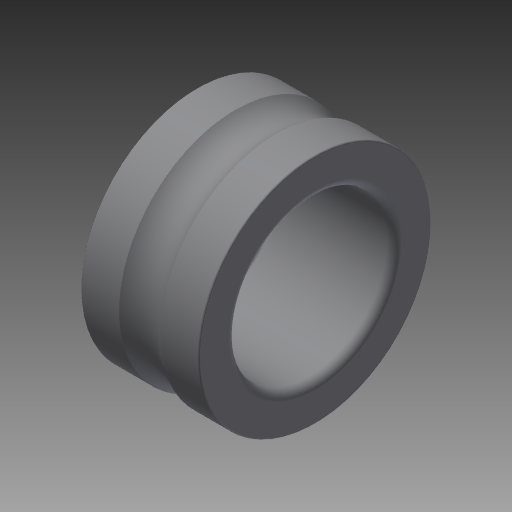
# Autodesk Inventor part: W 637/4 X_PART1
Saved by Autodesk Inventor 2019.1 (Build 231200000, 200)
## iProperties
Category: PARTsolutions
Company: SKF
Created: 2018-08-12
Part Number: W 637/4 X_PART1
Material: Allgemein
Catalog Web Link: www.cadenas.de
Description: -Deep groove ball bearings, stainless steel, single row
Vendor: SKF
Document SubType Name: Modeling
Designer: psadmin
Manufacturer: SKF
Mass: 0.0415935 g
Surface Area: 1.2092 cm^2
Volume: 0.0415935 cm^3
Density: 1 g/cm^3
Appearance: PSOLRGB-175-175-175
PSOL_IDENT_0: {$CADENAS_DATA\23d-libs\skf\bearings_units_and_housings\ball_bearings\deep_groove_ball_bearings\deep
PSOL_IDENT_1: _groove_ball_bearings_stainless_steel\bb1_004_104.prj},197 {VTYP=3D},{NB=W 637/4 X_PART1},{LINA=W 63
PSOL_IDENT_2: 7/4 X_PART1},{NN=BB1_004_104_PART1},{NOPRJ=TRUE},{DATE=13.07.2018 14:28:03},{GEOMDATE=26.07.2017 12:
PSOL_IDENT_3: 34:56},{VERSION=},{LINEID=77360},{WBVAR=},{WBNUMERIC=}  {NB=W 637/4 X_PART1},{LINA=W 637/4 X_PART1},
PSOL_IDENT_4: {KT=DUMMY},{PRODUCTID=},{DESIGNATION=W 637/4 X},{DD=4.000},{D=10.000},{B=3.000},{DD1=5.900},{DD2=MIN
PSOL_IDENT_5: },{D1=8.200},{D2=MIN},{R12A=0.200},{LOAD1=0.553},{LOAD2=0.245},{LOAD3=0.011},{SPEED1=80000},{SPEED2=
PSOL_IDENT_6: },{MASS=0.001},{PITCH=7.100},{DW=1.588},{Z=8.000},{II=1.000},{TYPEID=MIN},{YALG=2.95},{HALG=0.95},{H
PSOL_IDENT_7: ELP=0.9},{HELP2=500000007523733109938344427520},{YALG1=4.1},{HALG1=0.9},{TAXONOMY=2},{DESIGN=dgbbw},
PSOL_IDENT_8: {MAPPING=BCZ50,DESIGNATION|IRD01,DD|ORD10,D|BCW30,B|IRD30,DD1|ORD30,D1|ORD43,D2|IRD43,DD2|ORR20,R12A
PSOL_IDENT_9: |BCC02,LOAD1|BCC16,LOAD2|BCC12,LOAD3|BCC45,SPEED1|BCM01,MASS|BCD50,PITCH|RBD10,DW|BCN81,Z|BCN80,II},
PSOL_IDENT_10: {DESIGNLIST=dgbbw2z,dgbbw,dgbbw2rs},{SH=2.95},{SORT=DD},{RHELP=500000007523733109938344427520},{PIM=
PSOL_IDENT_11: W 637/4 X},{R12=0.2},{HIDE=MIN}
NT: Deep groove ball bearings, stainless steel, single row
NB: W 637/4 X_PART1
NBSYN: $DESIGNATION._PART1
LINA: W 637/4 X_PART1
SUPPLIER: SKF
ARTICLENO: W 637/4 X_PART1
BOMINFO: W 637/4 X_PART1
CREATOR: CADENAS GmbH
Title: W 637/4 X_PART1
Author: Cadenas PARTsolutions
Comments: Deep groove ball bearings, stainless steel, single row
Autodesk Inventor part; units mm, degrees
ref_plane "YZ Plane" through (0, 0, 0) normal (1, 0, 0) x (0, 1, 0)
ref_plane "XZ Plane" through (0, 0, 0) normal (0, 1, 0) x (-1, 0, 0)
ref_plane "XY Plane" through (0, 0, 0) normal (0, 0, 1) x (1, 0, 0)
sketch "Sketch_1" plane through (0, 0, 0) normal (0, 0, 1) x (1, 0, 0)
  line L0 (50, 0) -> (-50, 0)
  line L1 (0, 2.91) -> (0, 2.2)
  arc A0 (0, 2.2) -> (0.2, 2) centre (0.2, 2.2) ccw
  line L2 (0.2, 2) -> (2.8, 2)
  arc A1 (2.8, 2) -> (3, 2.2) centre (2.8, 2.2) ccw
  line L3 (3, 2.2) -> (3, 2.91)
  arc A2 (3, 2.91) -> (2.96, 2.95) centre (2.96, 2.91) ccw
  line L4 (2.96, 2.95) -> (2.02, 2.95)
  arc A3 (0.98, 2.95) -> (2.02, 2.95) centre (1.5, 3.55) ccw
  line L5 (0.98, 2.95) -> (0.04, 2.95)
  arc A4 (0.04, 2.95) -> (0, 2.91) centre (0.04, 2.91) ccw
  constraints: 12 end point, 10 point on circle, 5 centre point
revolve "Revolution1" add sketch "Sketch_1" angle 360 about axis through (50, 0, 0) along (1, 0, 0)
body "Solid1"
